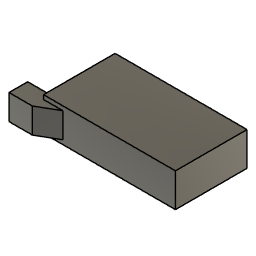
DogcomBattery (Autodesk Fusion 360 design; units mm, degrees)
Autodesk Fusion 360 part; units mm, degrees
sketch "Sketch1" plane through (0, 0, 0) normal (0, 0, 1) x (1, 0, 0)
  line L0 (0, 0) -> (56.6, 0)
  line L1 (56.6, 0) -> (56.6, 30.7)
  line L2 (56.6, 30.7) -> (0, 30.7)
  line L3 (0, 30.7) -> (0, 0)
  dimension "d1" = 56.6
  dimension "d2" = 30.7
  constraint horizontal L0
  constraint vertical L1
  constraint horizontal L2
  constraint vertical L3
  constraint coincident L0.start L3.end
  measures "d1" distance of L0.start L0.end
  measures "d2" distance of L0.start L2.end
extrude "Extrude1" add sketch "Sketch1" along normal blind 14.4
sketch "Sketch2" plane through (0, 0, 0) normal (-1, 0, 0) x (0, -1, 0)
  line L0 (-30.7, 0) -> (0, 0)
  line L1 (0, 14.4) -> (-30.7, 14.4)
  line L2 (-30.7, 14.4) -> (-30.7, 0)
  line L3 (4.8, 12.6) -> (-3.2, 12.6)
  line L4 (-3.2, 12.6) -> (-3.2, 1.8)
  line L5 (-3.2, 1.8) -> (4.8, 1.8)
  line L6 (4.8, 1.8) -> (4.8, 12.6)
  line L7 (0, 0) -> (0, 14.4)
  dimension "d9" = 8
  dimension "d10" = 3.2
  dimension "d11" = 1.8
  dimension "d12" = 1.8
  constraint horizontal L3
  constraint vertical L4
  constraint horizontal L5
  constraint vertical L6
  measures "d9" distance of L3.start L3.end
  measures "d10" distance of L4 L7
  measures "d11" distance of L5 L0.end
  measures "d12" distance of L3 L1.start
extrude "Extrude2" add sketch "Sketch2" along normal blind 10 contours L3 L5 L6 L7 | L3 L4 L5 L7
chamfer "Chamfer1" distance 4.8 angle 60 1 edges at (0, 0, 7.2) measured on face at (0, -1.6, 5.4)
equation "d12 = d11"
